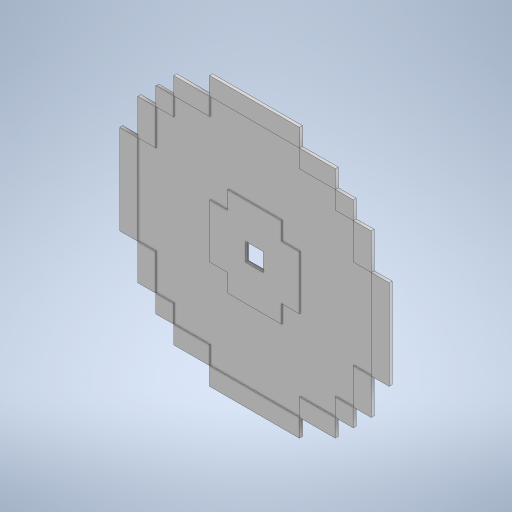
# Autodesk Inventor part: Disc 4
Saved by Autodesk Inventor 2024 (Build 280153000, 153)
## iProperties
Created: 2024-02-02
Part Number: Disc 4
Material: Generic
Document SubType Name: Modeling
Designer: newic
Density: 1 g/cm^3
Appearance: Default
Author: newic
Autodesk Inventor part; units mm, degrees
ref_plane "YZ Plane" through (0, 0, 0) normal (1, 0, 0) x (0, 1, 0)
ref_plane "XZ Plane" through (0, 0, 0) normal (0, 1, 0) x (-1, 0, 0)
ref_plane "XY Plane" through (0, 0, 0) normal (0, 0, 1) x (1, 0, 0)
sketch "Sketch1" plane through (0, 0, 0) normal (0, 0, 1) x (1, 0, 0)
  circle A0 centre (0, 0) radius 152.4
  circle A1 centre (0, 0) radius 5.5
  dimension "d0" = 304.8
  dimension "d1" = 11
  constraints: 2 centre point, 2 coincident
  measures "d0" diameter of A0
  measures "d1" diameter of A1
extrude "Extrusion1" add sketch "Sketch1" along normal blind 2.2
fillet "Fillet1" radius 1.1 2 edges at (-152.4, 0, 0) (-152.4, 0, 2.2)
sketch "Sketch2" plane through (0, 0, 2.2) normal (0, 0, 1) x (1, 0, 0)
  line L0 (206.2137, 42.4617) -> (289.822, 42.4617) construction
  line L1 (289.822, 42.4617) -> (289.822, -13.3654) construction
  line L2 (289.822, -13.3654) -> (206.2137, -13.3654) construction
  line L3 (206.2137, -13.3654) -> (206.2137, 42.4617) construction
  line L4 (9.525, 9.525) -> (-9.525, 9.525)
  line L5 (-9.525, 9.525) -> (-9.525, -9.525)
  line L6 (-9.525, -9.525) -> (9.525, -9.525)
  line L7 (9.525, -9.525) -> (9.525, 9.525)
  line L8 (-123.825, 47.625) -> (-104.775, 47.625)
  line L9 (-123.825, -47.625) -> (-142.875, -47.625)
  line L10 (-123.825, -47.625) -> (-104.775, -47.625)
  line L11 (0, 9.525) -> (0, -9.525)
  line L12 (-9.525, 0) -> (9.525, 0)
  line L13 (0, 0) -> (-4.1012, 3.8959)
  line L14 (-142.875, 28.575) -> (-123.825, 28.575)
  line L15 (-123.825, 28.575) -> (-123.825, 9.525)
  line L16 (-123.825, 9.525) -> (-142.875, 9.525)
  line L17 (-142.875, 9.525) -> (-142.875, 28.575)
  line L18 (-142.875, -9.525) -> (-123.825, -9.525)
  line L19 (-123.825, -9.525) -> (-123.825, 9.525)
  line L20 (-142.875, 9.525) -> (-142.875, -9.525)
  line L21 (-123.825, -47.625) -> (-123.825, -28.575)
  line L22 (-123.825, -28.575) -> (-142.875, -28.575)
  line L23 (-142.875, -28.575) -> (-142.875, -47.625)
  line L24 (-123.825, -9.525) -> (-123.825, -28.575)
  line L25 (-142.875, -28.575) -> (-142.875, -9.525)
  line L26 (-123.825, 47.625) -> (-104.775, 47.625)
  line L27 (-104.775, 47.625) -> (-104.775, 66.675)
  line L28 (-104.775, 66.675) -> (-123.825, 66.675)
  line L29 (-123.825, 66.675) -> (-123.825, 47.625)
  line L30 (-123.825, -47.625) -> (-104.775, -47.625)
  line L31 (-104.775, -47.625) -> (-104.775, -66.675)
  line L32 (-104.775, -66.675) -> (-123.825, -66.675)
  line L33 (-123.825, -66.675) -> (-123.825, -47.625)
  circle A0 centre (0, 0) radius 350.7035
  line L34 (-123.825, -85.725) -> (-104.775, -85.725)
  line L35 (-123.825, -85.725) -> (-104.775, -85.725)
  line L36 (-104.775, -85.725) -> (-104.775, -66.675)
  line L37 (-123.825, -66.675) -> (-123.825, -85.725)
  line L38 (-123.825, 85.725) -> (-104.775, 85.725)
  line L39 (-123.825, 85.725) -> (-104.775, 85.725)
  line L40 (-104.775, 85.725) -> (-104.775, 66.675)
  line L41 (-123.825, 66.675) -> (-123.825, 85.725)
  line L42 (-104.775, 85.725) -> (-85.725, 85.725)
  line L43 (-85.725, 85.725) -> (-85.725, 104.775)
  line L44 (-85.725, 104.775) -> (-104.775, 104.775)
  line L45 (-104.775, 104.775) -> (-104.775, 85.725)
  line L46 (-104.775, -85.725) -> (-85.725, -85.725)
  line L47 (-85.725, -85.725) -> (-85.725, -104.775)
  line L48 (-85.725, -104.775) -> (-104.775, -104.775)
  line L49 (-104.775, -104.775) -> (-104.775, -85.725)
  line L50 (-85.725, 104.775) -> (-66.675, 104.775)
  line L51 (-66.675, 104.775) -> (-66.675, 123.825)
  line L52 (-66.675, 123.825) -> (-85.725, 123.825)
  line L53 (-85.725, 123.825) -> (-85.725, 104.775)
  line L54 (-85.725, -104.775) -> (-66.675, -104.775)
  line L55 (-66.675, -104.775) -> (-66.675, -123.825)
  line L56 (-66.675, -123.825) -> (-85.725, -123.825)
  line L57 (-85.725, -123.825) -> (-85.725, -104.775)
  line L58 (-142.875, 28.575) -> (-123.825, 28.575)
  line L59 (-123.825, 28.575) -> (-123.825, 47.625)
  line L60 (-123.825, 47.625) -> (-142.875, 47.625)
  line L61 (-142.875, 47.625) -> (-142.875, 28.575)
  line L62 (-47.625, 104.775) -> (-66.675, 104.775)
  line L63 (-66.675, 123.825) -> (-47.625, 123.825)
  line L64 (-47.625, 123.825) -> (-47.625, 104.775)
  line L65 (-47.625, -104.775) -> (-66.675, -104.775)
  line L66 (-66.675, -123.825) -> (-47.625, -123.825)
  line L67 (-47.625, -123.825) -> (-47.625, -104.775)
  line L68 (-47.625, 123.825) -> (-28.575, 123.825)
  line L69 (-28.575, 123.825) -> (-28.575, 142.875)
  line L70 (-28.575, 142.875) -> (-47.625, 142.875)
  line L71 (-47.625, 142.875) -> (-47.625, 123.825)
  line L72 (-47.625, -123.825) -> (-28.575, -123.825)
  line L73 (-28.575, -123.825) -> (-28.575, -142.875)
  line L74 (-28.575, -142.875) -> (-47.625, -142.875)
  line L75 (-47.625, -142.875) -> (-47.625, -123.825)
  line L76 (-9.525, 123.825) -> (-28.575, 123.825)
  line L77 (-28.575, 142.875) -> (-9.525, 142.875)
  line L78 (-9.525, 142.875) -> (-9.525, 123.825)
  line L79 (-9.525, -123.825) -> (-28.575, -123.825)
  line L80 (-28.575, -142.875) -> (-9.525, -142.875)
  line L81 (-9.525, -142.875) -> (-9.525, -123.825)
  line L82 (9.525, 123.825) -> (9.525, 142.875)
  line L83 (9.525, -123.825) -> (9.525, -142.875)
  line L84 (-9.525, 123.825) -> (9.525, 123.825)
  line L85 (9.525, 142.875) -> (-9.525, 142.875)
  line L86 (-9.525, -123.825) -> (9.525, -123.825)
  line L87 (9.525, -142.875) -> (-9.525, -142.875)
  line L88 (9.525, 9.525) -> (9.525, -9.525)
  line L89 (-9.525, 9.525) -> (9.525, 9.525)
  line L90 (9.525, -9.525) -> (-9.525, -9.525)
  line L91 (-9.525, -9.525) -> (-9.525, 9.525)
  line L92 (123.825, 47.625) -> (104.775, 47.625)
  line L93 (123.825, -47.625) -> (104.775, -47.625)
  line L94 (123.825, -47.625) -> (142.875, -47.625)
  line L95 (9.525, 0) -> (-9.525, 0)
  line L96 (0, 0) -> (4.1012, 3.8959)
  line L97 (142.875, 28.575) -> (123.825, 28.575)
  line L98 (123.825, 28.575) -> (123.825, 9.525)
  line L99 (123.825, 9.525) -> (142.875, 9.525)
  line L100 (142.875, 9.525) -> (142.875, 28.575)
  line L101 (123.825, -9.525) -> (123.825, 9.525)
  line L102 (142.875, -9.525) -> (123.825, -9.525)
  line L103 (142.875, 9.525) -> (142.875, -9.525)
  line L104 (123.825, -9.525) -> (123.825, -28.575)
  line L105 (123.825, -47.625) -> (123.825, -28.575)
  line L106 (142.875, -28.575) -> (142.875, -9.525)
  line L107 (123.825, -28.575) -> (142.875, -28.575)
  line L108 (142.875, -28.575) -> (142.875, -47.625)
  line L109 (123.825, 47.625) -> (104.775, 47.625)
  line L110 (104.775, 47.625) -> (104.775, 66.675)
  line L111 (104.775, 66.675) -> (123.825, 66.675)
  line L112 (123.825, 66.675) -> (123.825, 47.625)
  line L113 (123.825, -47.625) -> (104.775, -47.625)
  line L114 (104.775, -47.625) -> (104.775, -66.675)
  line L115 (104.775, -66.675) -> (123.825, -66.675)
  line L116 (123.825, -66.675) -> (123.825, -47.625)
  line L117 (123.825, -85.725) -> (104.775, -85.725)
  line L118 (104.775, -85.725) -> (104.775, -66.675)
  line L119 (123.825, -66.675) -> (123.825, -85.725)
  line L120 (123.825, -85.725) -> (104.775, -85.725)
  line L121 (123.825, 85.725) -> (104.775, 85.725)
  line L122 (104.775, 85.725) -> (104.775, 66.675)
  line L123 (123.825, 85.725) -> (104.775, 85.725)
  line L124 (123.825, 66.675) -> (123.825, 85.725)
  line L125 (104.775, 85.725) -> (85.725, 85.725)
  line L126 (85.725, 85.725) -> (85.725, 104.775)
  line L127 (85.725, 104.775) -> (104.775, 104.775)
  line L128 (104.775, 104.775) -> (104.775, 85.725)
  line L129 (104.775, -85.725) -> (85.725, -85.725)
  line L130 (85.725, -85.725) -> (85.725, -104.775)
  line L131 (85.725, -104.775) -> (104.775, -104.775)
  line L132 (104.775, -104.775) -> (104.775, -85.725)
  line L133 (85.725, 104.775) -> (66.675, 104.775)
  line L134 (66.675, 104.775) -> (66.675, 123.825)
  line L135 (66.675, 123.825) -> (85.725, 123.825)
  line L136 (85.725, 123.825) -> (85.725, 104.775)
  line L137 (85.725, -104.775) -> (66.675, -104.775)
  line L138 (66.675, -104.775) -> (66.675, -123.825)
  line L139 (66.675, -123.825) -> (85.725, -123.825)
  line L140 (85.725, -123.825) -> (85.725, -104.775)
  line L141 (142.875, 28.575) -> (123.825, 28.575)
  line L142 (123.825, 28.575) -> (123.825, 47.625)
  line L143 (123.825, 47.625) -> (142.875, 47.625)
  line L144 (142.875, 47.625) -> (142.875, 28.575)
  line L145 (47.625, 104.775) -> (66.675, 104.775)
  line L146 (66.675, 123.825) -> (47.625, 123.825)
  line L147 (47.625, 123.825) -> (47.625, 104.775)
  line L148 (47.625, -104.775) -> (66.675, -104.775)
  line L149 (47.625, -123.825) -> (47.625, -104.775)
  line L150 (66.675, -123.825) -> (47.625, -123.825)
  line L151 (47.625, 123.825) -> (28.575, 123.825)
  line L152 (28.575, 123.825) -> (28.575, 142.875)
  line L153 (28.575, 142.875) -> (47.625, 142.875)
  line L154 (47.625, 142.875) -> (47.625, 123.825)
  line L155 (47.625, -123.825) -> (28.575, -123.825)
  line L156 (28.575, -123.825) -> (28.575, -142.875)
  line L157 (28.575, -142.875) -> (47.625, -142.875)
  line L158 (47.625, -142.875) -> (47.625, -123.825)
  line L159 (9.525, 123.825) -> (28.575, 123.825)
  line L160 (9.525, 142.875) -> (9.525, 123.825)
  line L161 (28.575, 142.875) -> (9.525, 142.875)
  line L162 (9.525, -142.875) -> (9.525, -123.825)
  line L163 (9.525, -123.825) -> (28.575, -123.825)
  line L164 (28.575, -142.875) -> (9.525, -142.875)
  line L165 (-9.525, 123.825) -> (-9.525, 142.875)
  line L166 (9.525, 123.825) -> (-9.525, 123.825)
  line L167 (-9.525, 142.875) -> (9.525, 142.875)
  line L168 (-9.525, -123.825) -> (-9.525, -142.875)
  line L169 (9.525, -123.825) -> (-9.525, -123.825)
  line L170 (-9.525, -142.875) -> (9.525, -142.875)
  point P0 (-123.825, -9.525)
  point P1 (-123.825, -47.625)
  point P2 (-123.825, -85.725)
  point P3 (123.825, -9.525)
  point P4 (123.825, -47.625)
  point P5 (123.825, -85.725)
  dimension "d22" = 19.05
  dimension "d23" = 19.05
  dimension "d29" = 19.05
  dimension "d30" = 19.05
  dimension "d35" = 19.05
  dimension "d36" = 19.05
  dimension "d67" = 19.05
  dimension "d68" = 19.05
  dimension "d69" = 19.05
  dimension "d70" = 19.05
  dimension "d71" = 19.05
  dimension "d72" = 19.05
  dimension "d73" = 19.05
  dimension "d74" = 19.05
  dimension "d77" = 19.05
  dimension "d78" = 19.05
  dimension "d79" = 19.05
  dimension "d80" = 19.05
  constraints: 334 end point, 98 symmetric about line, 20 parallel, 10 horizontal, 10 perpendicular, 5 midpoint, 2 coincident, 1 centre point, 2 other
  measures "d22" distance of L15.end L16.end
  measures "d23" distance of L15.start L15.end
  measures "d29" distance of L28.end L27.end
  measures "d30" distance of L27.end L26.end
  measures "d35" distance of L31.end L32.end
  measures "d36" distance of L30.end L31.end
  measures "d67" distance of L44.end L43.end
  measures "d68" distance of L43.end L42.end
  measures "d69" distance of L47.end L48.end
  measures "d70" distance of L46.end L47.end
  measures "d71" distance of L52.end L51.end
  measures "d72" distance of L51.end L50.end
  measures "d73" distance of L55.end L56.end
  measures "d74" distance of L54.end L55.end
  measures "d77" distance of L70.end L69.end
  measures "d78" distance of L69.end L68.end
  measures "d79" distance of L73.end L74.end
  measures "d80" distance of L72.end L73.end
extrude "Extrusion2" cut sketch "Sketch2" against normal blind 25.4
sketch "Sketch3" plane through (0, 0, 2.2) normal (0, 0, 1) x (1, 0, 0)
  line L0 (-123.825, 47.625) -> (-142.875, 47.625) projected
  line L1 (-142.875, 47.625) -> (-123.825, 47.625)
  line L2 (-123.825, 47.625) -> (-123.825, -47.625)
  line L3 (-123.825, -47.625) -> (-142.875, -47.625)
  line L4 (-142.875, -47.625) -> (-142.875, 47.625)
  line L5 (-123.825, -47.625) -> (-123.825, -85.725) projected
  line L6 (-123.825, -85.725) -> (-104.775, -85.725) projected
  line L7 (-123.825, -47.625) -> (-104.775, -47.625)
  line L8 (-104.775, -47.625) -> (-104.775, -85.725)
  line L9 (-104.775, -85.725) -> (-123.825, -85.725)
  line L10 (-123.825, -85.725) -> (-123.825, -47.625)
  line L11 (-104.775, -104.775) -> (-85.725, -104.775) projected
  line L12 (-104.775, -85.725) -> (-85.725, -85.725)
  line L13 (-85.725, -85.725) -> (-85.725, -104.775)
  line L14 (-85.725, -104.775) -> (-104.775, -104.775)
  line L15 (-104.775, -104.775) -> (-104.775, -85.725)
  line L16 (-85.725, -104.775) -> (-47.625, -104.775)
  line L17 (-47.625, -104.775) -> (-47.625, -123.825)
  line L18 (-47.625, -123.825) -> (-85.725, -123.825)
  line L19 (-85.725, -123.825) -> (-85.725, -104.775)
  line L20 (-47.625, -142.875) -> (47.625, -142.875) projected
  line L21 (-47.625, -123.825) -> (47.625, -123.825)
  line L22 (47.625, -123.825) -> (47.625, -142.875)
  line L23 (47.625, -142.875) -> (-47.625, -142.875)
  line L24 (-47.625, -142.875) -> (-47.625, -123.825)
  line L25 (-104.775, 85.725) -> (-123.825, 85.725) projected
  line L26 (-104.775, 85.725) -> (-123.825, 85.725)
  line L27 (-123.825, 85.725) -> (-123.825, 47.625)
  line L28 (-123.825, 47.625) -> (-104.775, 47.625)
  line L29 (-104.775, 47.625) -> (-104.775, 85.725)
  line L30 (-85.725, 105.1059) -> (-104.775, 105.1059)
  line L31 (-104.775, 105.1059) -> (-104.775, 85.725)
  line L32 (-104.775, 85.725) -> (-85.725, 85.725)
  line L33 (-85.725, 85.725) -> (-85.725, 105.1059)
  line L34 (-47.625, 123.825) -> (-85.725, 123.825)
  line L35 (-85.725, 123.825) -> (-85.725, 105.1059)
  line L36 (-85.725, 105.1059) -> (-47.625, 105.1059)
  line L37 (-47.625, 105.1059) -> (-47.625, 123.825)
  line L38 (47.625, 123.825) -> (47.625, 142.875) projected
  line L39 (47.625, 142.875) -> (-47.625, 142.875)
  line L40 (-47.625, 142.875) -> (-47.625, 123.825)
  line L41 (-47.625, 123.825) -> (47.625, 123.825)
  line L42 (47.625, 123.825) -> (47.625, 142.875)
  line L43 (85.725, 104.775) -> (85.725, 123.825) projected
  line L44 (47.625, 123.825) -> (85.725, 123.825)
  line L45 (85.725, 123.825) -> (85.725, 104.775)
  line L46 (85.725, 104.775) -> (47.625, 104.775)
  line L47 (47.625, 104.775) -> (47.625, 123.825)
  line L48 (104.775, 85.725) -> (104.775, 104.775) projected
  line L49 (85.725, 104.775) -> (104.775, 104.775)
  line L50 (104.775, 104.775) -> (104.775, 85.725)
  line L51 (104.775, 85.725) -> (85.725, 85.725)
  line L52 (85.725, 85.725) -> (85.725, 104.775)
  line L53 (123.825, 85.725) -> (123.825, 47.625) projected
  line L54 (104.775, 85.725) -> (123.825, 85.725)
  line L55 (123.825, 85.725) -> (123.825, 47.625)
  line L56 (123.825, 47.625) -> (104.775, 47.625)
  line L57 (104.775, 47.625) -> (104.775, 85.725)
  line L58 (123.825, 47.625) -> (142.875, 47.625)
  line L59 (142.875, 47.625) -> (142.875, -47.625)
  line L60 (142.875, -47.625) -> (123.825, -47.625)
  line L61 (123.825, -47.625) -> (123.825, 47.625)
  line L62 (123.825, -47.625) -> (104.775, -47.625)
  line L63 (104.775, -47.625) -> (104.775, -85.725)
  line L64 (104.775, -85.725) -> (123.825, -85.725)
  line L65 (123.825, -85.725) -> (123.825, -47.625)
  line L66 (104.775, -85.725) -> (85.725, -85.725)
  line L67 (85.725, -85.725) -> (85.725, -104.775)
  line L68 (85.725, -104.775) -> (104.775, -104.775)
  line L69 (104.775, -104.775) -> (104.775, -85.725)
  line L70 (47.625, -123.825) -> (85.725, -123.825) projected
  line L71 (85.725, -104.775) -> (47.625, -104.775)
  line L72 (47.625, -104.775) -> (47.625, -123.825)
  line L73 (47.625, -123.825) -> (85.725, -123.825)
  line L74 (85.725, -123.825) -> (85.725, -104.775)
  line L75 (-9.525, 9.525) -> (-9.525, -9.525) projected
  line L76 (-9.525, -9.525) -> (-28.575, -9.525)
  line L77 (-28.575, -9.525) -> (-28.575, -28.575)
  line L78 (-28.575, -28.575) -> (-9.525, -28.575)
  line L79 (-9.525, -28.575) -> (-9.525, -9.525)
  line L80 (9.525, 9.525) -> (-9.525, 9.525) projected
  line L81 (9.525, 9.525) -> (28.575, 9.525)
  line L82 (28.575, 9.525) -> (28.575, 28.575)
  line L83 (28.575, 28.575) -> (9.525, 28.575)
  line L84 (9.525, 28.575) -> (9.525, 9.525)
  line L85 (-28.575, -28.575) -> (28.575, -28.575)
  line L86 (28.575, -28.575) -> (28.575, 28.575)
  line L87 (28.575, 28.575) -> (-28.575, 28.575)
  line L88 (-28.575, 28.575) -> (-28.575, -28.575)
  line L89 (-28.575, -28.575) -> (-47.625, -28.575)
  line L90 (-47.625, -28.575) -> (-47.625, 28.575)
  line L91 (-47.625, 28.575) -> (-28.575, 28.575)
  line L92 (-28.575, 28.575) -> (-28.575, -28.575)
  line L93 (28.575, -28.575) -> (47.625, -28.575)
  line L94 (47.625, -28.575) -> (47.625, 28.575)
  line L95 (47.625, 28.575) -> (28.575, 28.575)
  line L96 (28.575, 28.575) -> (28.575, -28.575)
  line L97 (28.575, -28.575) -> (-28.575, -28.575)
  line L98 (-28.575, -28.575) -> (-28.575, -47.625)
  line L99 (-28.575, -47.625) -> (28.575, -47.625)
  line L100 (28.575, -47.625) -> (28.575, -28.575)
  line L101 (-28.575, 28.575) -> (28.575, 28.575)
  line L102 (28.575, 28.575) -> (28.575, 47.625)
  line L103 (28.575, 47.625) -> (-28.575, 47.625)
  line L104 (-28.575, 47.625) -> (-28.575, 28.575)
  line L105 (-9.525, 9.525) -> (9.525, 9.525)
  line L106 (9.525, 9.525) -> (9.525, -9.525)
  line L107 (9.525, -9.525) -> (-9.525, -9.525)
  line L108 (-9.525, -9.525) -> (-9.525, 9.525)
  point P0 (0, 0)
  dimension "d89" = 19.05
  dimension "d90" = 19.05
  dimension "d91" = 19.05
  dimension "d92" = 19.05
  dimension "d93" = 19.05
  constraints: 192 end point, 48 parallel, 24 horizontal, 24 perpendicular, 7 point on line
  measures "d89" distance of L78.end L77.end
  measures "d90" distance of L77.end L76.end
  measures "d91" distance of L83.end L82.end
  measures "d92" distance of L82.end L81.end
  measures "d93" distance of L90.end L91.end
extrude "Extrusion3" add sketch "Sketch3" along normal blind 0.9 contours L2 L3 L4 L0 | L27 L25 L29 L28 | L7 L8 L6 L5 | L31 L30 L33 L32 | L12 L13 L11 L15 | L35 L34 L37 L36 | L16 L17 L18 L19 | L40 L39 L38 L41 | L21 L22 L20 L24 | L44 L43 L46 L47 | L72 L71 L74 L70 | L49 L48 L51 L52 | L67 L66 L69 L68 | L54 L53 L56 L57 | L63 L62 L65 L64 | L58 L59 L60 L61 | L75 L76 L88 L87 L84 L80 | L79 L78 L77 L76 | L107 L106 L81 L86 L85 L79 | L84 L83 L82 L81 | L77 L89 L90 L91 L88 | L85 L100 L99 L98 L78 | L82 L95 L94 L93 L86 | L87 L104 L103 L102 L83
body "Solid1"
